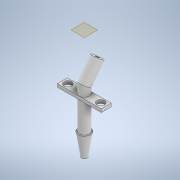
# Autodesk Inventor part: Düse
Saved by Autodesk Inventor 2021 (Build 250183000, 183)
## iProperties
Created: 2021-12-20
Part Number: Düse
Material: Generisch
Document SubType Name: Modeling
Designer: stroh
Density: 1 g/cm^3
Appearance: Vorgabe
Author: stroh
Autodesk Inventor part; units mm, degrees
ref_plane "YZ Plane" through (0, 0, 0) normal (1, 0, 0) x (0, 1, 0)
ref_plane "XY Plane" through (0, 0, 0) normal (0, 0, 1) x (1, 0, 0)
sketch "Skizze1" plane through (0, 0, 0) normal (0, 0, 1) x (1, 0, 0)
  line L0 (-3.3, 0) -> (0.55, 0) projected
  line L1 (0, -6) -> (0, 36) projected
  line L2 (-1.25, 0) -> (-0.75, 0)
  line L3 (-0.75, 0) -> (-0.75, 30)
  line L4 (-0.75, 30) -> (-2.25, 30)
  line L5 (-2.25, 30) -> (-2.25, 10)
  line L6 (-2.25, 10) -> (-2.75, 10)
  line L7 (-2.75, 10) -> (-1.25, 0)
  point P0 (0, 0)
  dimension "d0" = 1.5
  dimension "d1" = 0.5
  dimension "d2" = 0.5
  dimension "d3" = 0.75
  dimension "d6" = 30
  dimension "d7" = 10
  constraints: 12 end point, 3 perpendicular, 2 point on line, 1 vertical
  measures "d0" distance of L3.end L4.end
  measures "d1" distance of L5.end L6.end
  measures "d2" distance of L2.end L2.start
  measures "d3" distance from line of L1 L3.end
  measures "d6" distance from line of L2.end L4
  measures "d7" distance from line of L0 L5.end
revolve "Umdrehung1" add sketch "Skizze1" angle 360 about axis through (0, -10, 0) along (0, 1, 0)
ref_plane "Arbeitsebene1" through (0, 50, 0) normal (0, 1, 0) x (-1, 0, 0)
sketch "Skizze3" plane through (0, 0, 0) normal (1, 0, 0) x (0, 1, 0)
  line L0 (30, -2.25) -> (30, 2.25) projected
  line L1 (30, 2.25) -> (26.6518, -2.25)
  line L2 (10, -2.25) -> (30, -2.25) projected
  line L3 (30, 2.25) -> (30, -2.25)
  line L4 (30, -2.25) -> (26.6518, -2.25)
  point P0 (0, 0)
  constraints: 6 end point, 1 perpendicular, 1 point on line, 1 vertical
extrude "Extrusion1" cut sketch "Skizze3" against normal mid plane 10
sketch "Skizze4" plane through (0, 28.3259, 0) normal (0, 0.8022892, -0.5969355) x (1, 0, 0)
  ellipse E0 centre (0, 0) end of major axis (0, -2.8045) minor radius 2.25 projected
  ellipse E1 centre (0, 0) end of major axis (0, -2.8045) minor radius 2.25
  ellipse E2 centre (0, 0) end of major axis (0, -0.9255) minor radius 0.7538
  point P0 (0, 16.9087)
  constraints: 2 coincident, 5 other
extrude "Extrusion2" add sketch "Skizze4" along normal blind 10
sketch "Skizze5" plane through (0, 0, 0) normal (1, 0, 0) x (0, 1, 0)
  line L0 (25, 2.25) -> (23.5, 2.25)
  line L1 (23.5, 2.25) -> (23.5, -2.25)
  line L2 (23.5, -2.25) -> (25, -2.25)
  line L3 (25, -2.25) -> (25, 2.25)
  line L4 (-7.6046, 0) -> (45.6275, 0) projected
  line L5 (0, -10.4132) -> (0, 4.9439) projected
  point P0 (0, 0)
  dimension "d23" = 4.5
  dimension "d24" = 2.25
  dimension "d25" = 25
  dimension "d26" = 1.5
  constraints: 8 end point, 2 parallel, 1 horizontal, 1 perpendicular
  measures "d23" distance of L0.start L2.end
  measures "d24" distance from line of L4 L2.end
  measures "d25" distance between parallel lines of L5 L3
  measures "d26" distance of L1.end L2.end
extrude "Extrusion3" add sketch "Skizze5" along normal mid plane 20
sketch "Skizze6" plane through (0, 0, 0) normal (0, -1, 0) x (1, 0, 0)
  circle A0 centre (0, 0) radius 0.75
  constraints: 1 centre point, 1 coincident
extrude "Extrusion4" cut sketch "Skizze6" against normal blind 27
sketch "Skizze7" plane through (0, 25, 2.25) normal (0, 1, 0) x (1, 0, 0)
  circle A0 centre (7.5, 2.25) radius 1.75
  circle A1 centre (-7.5, 2.25) radius 1.75
  line L0 (10, 4.5) -> (10, 0) projected
  point P0 (0, 2.25)
  dimension "d31" = 3.5
  dimension "d32" = 3.5
  dimension "d33" = 15
  dimension "d34" = 2.5
  constraints: 2 centre point
  measures "d31" diameter of A0
  measures "d32" diameter of A1
  measures "d33" distance of A0.centre A1.centre
  measures "d34" distance from line of L0 A0.centre
extrude "Extrusion5" cut sketch "Skizze7" against normal blind 5
